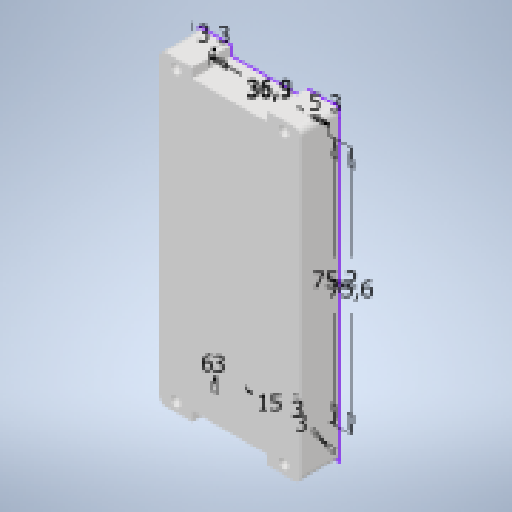
# Autodesk Inventor part: fast_akkum2
Saved by Autodesk Inventor 2023 (Build 270158000, 158)
## iProperties
Created: 2026-02-17
Part Number: fast_akkum2
Material: Типовые
Document SubType Name: Modeling
Designer: garin
Density: 1 g/cm^3
Appearance: По умолчанию
Author: garin
Autodesk Inventor part; units mm, degrees
ref_plane "YZ Plane" through (0, 0, 0) normal (1, 0, 0) x (0, 1, 0)
ref_plane "XZ Plane" through (0, 0, 0) normal (0, 1, 0) x (-1, 0, 0)
ref_plane "XY Plane" through (0, 0, 0) normal (0, 0, 1) x (1, 0, 0)
sketch "Эскиз1" plane through (0, 0, 0) normal (0, 0, 1) x (1, 0, 0)
  line L0 (-18.25, -37.6) -> (18.25, -37.6)
  line L1 (18.25, -37.6) -> (18.25, 37.6)
  line L2 (18.25, 37.6) -> (-18.25, 37.6)
  line L3 (-18.25, 37.6) -> (-18.25, -37.6)
  line L4 (-18.25, 0) -> (18.25, 0) construction
  line L5 (0, 37.6) -> (0, -37.6) construction
  line L6 (-18.45, -37.8) -> (18.45, -37.8)
  line L7 (18.45, -37.8) -> (18.45, 37.8)
  line L8 (18.45, 37.8) -> (-18.45, 37.8)
  line L9 (-18.45, 37.8) -> (-18.45, -37.8)
  line L10 (-7.5, -37.8) -> (7.5, -37.8)
  line L11 (7.5, -37.8) -> (7.5, -40.8)
  line L12 (7.5, -40.8) -> (-7.5, -40.8)
  line L13 (-7.5, -40.8) -> (-7.5, -37.8)
  line L14 (-18.45, -37.8) -> (-18.45, -43.8)
  line L15 (-18.45, -43.8) -> (18.45, -43.8)
  line L16 (18.45, -43.8) -> (18.45, -37.8)
  line L17 (-18.45, 43.8) -> (18.45, 43.8)
  line L18 (-18.45, 37.8) -> (-18.45, 43.8)
  line L19 (18.45, 43.8) -> (18.45, 37.8)
  line L20 (-18.45, -43.8) -> (-21.45, -43.8)
  line L21 (-21.45, -43.8) -> (-21.45, 43.8)
  line L22 (-21.45, 43.8) -> (-18.45, 43.8)
  line L23 (-18.45, 43.8) -> (-18.45, -43.8)
  line L24 (21.45, 43.8) -> (18.45, 43.8)
  line L25 (18.45, 37.8) -> (18.45, 43.8)
  line L26 (18.45, 43.8) -> (18.45, -43.8)
  line L27 (21.45, -43.8) -> (21.45, 43.8)
  line L28 (-7.5, 40.8) -> (-7.5, 37.8)
  line L29 (7.5, 40.8) -> (-7.5, 40.8)
  line L30 (7.5, 37.8) -> (7.5, 40.8)
  line L31 (-21.45, -43.8) -> (-11.45, -43.8)
  line L32 (18.45, -43.8) -> (21.45, -43.8)
  line L33 (21.45, -43.8) -> (11.45, -43.8)
  line L34 (16.45, 46.7) -> (21.45, 46.7)
  line L35 (16.45, 46.7) -> (11.45, 46.7)
  line L36 (11.45, 46.7) -> (11.45, 43.8)
  line L37 (21.45, 46.7) -> (21.45, 43.8)
  line L38 (11.45, 43.8) -> (16.45, 43.8)
  line L39 (-11.45, 46.7) -> (-11.45, 43.8)
  line L40 (-16.45, 46.7) -> (-11.45, 46.7)
  line L41 (-16.45, 46.7) -> (-21.45, 46.7)
  line L42 (-21.45, 46.7) -> (-21.45, 43.8)
  line L43 (-16.45, -46.7) -> (-21.45, -46.7)
  line L44 (-21.45, -46.7) -> (-21.45, -43.8)
  line L45 (-16.45, -46.7) -> (-11.45, -46.7)
  line L46 (-11.45, -46.7) -> (-11.45, -43.8)
  line L47 (11.45, -46.7) -> (11.45, -43.8)
  line L48 (16.45, -46.7) -> (11.45, -46.7)
  line L49 (16.45, -46.7) -> (21.45, -46.7)
  line L50 (21.45, -46.7) -> (21.45, -43.8)
  circle A0 centre (16.45, -43.8) radius 1.5
  circle A1 centre (-16.45, -43.8) radius 1.5
  circle A2 centre (16.45, 43.8) radius 1.5
  circle A3 centre (-16.45, 43.8) radius 1.5
  line L51 (0, 0) -> (-14.3, 0) construction
  line L52 (-14.3, 0) -> (-14.3, 38.8) construction
  line L53 (-14.3, 38.8) -> (0, 38.8) construction
  line L54 (0, 38.8) -> (0, 0) construction
  circle A4 centre (-14.3, 38.8) radius 1.25
  point P0 (-1.9914, -32.8601)
  point P1 (0, -37.8)
  point P2 (-15.05, 37.8)
  point P3 (-13.55, 37.8)
  dimension "d0" = 36.5
  dimension "d1" = 75.2
  dimension "d2" = 36.9
  dimension "d3" = 75.6
  dimension "d4" = 15
  dimension "d5" = 3
  dimension "d6" = 6
  dimension "d7" = 3
  dimension "d8" = 5
  dimension "d10" = 3
  dimension "d11" = 3
  dimension "d12" = 3
  dimension "d13" = 3
  dimension "d19" = 14.3
  dimension "d20" = 38.8
  dimension "d21" = 2.5
  constraints: 110 end point, 20 symmetric about line, 10 parallel, 9 perpendicular, 7 horizontal, 6 midpoint, 6 point on line, 5 centre point, 2 coincident, 2 vertical
  measures "d0" distance of L2.end L1.end
  measures "d1" distance of L1.end L0.end
  measures "d2" distance of L9.start L7.end
  measures "d3" distance of L7.end L7.start
  measures "d4" distance of L11.end L13.start
  measures "d5" distance of L10.end L11.end
  measures "d6" distance of L9.end L23.end
  measures "d7" distance of L21.end L23.start
  measures "d8" distance of L36.end L38.end
  measures "d10" diameter of A0
  measures "d11" diameter of A1
  measures "d12" diameter of A2
  measures "d13" diameter of A3
  measures "d19" distance of L52.end L53.end
  measures "d20" distance of L51.end L52.end
  measures "d21" diameter of A4
extrude "Выдавливание1" add sketch "Эскиз1" along normal blind 12 contours A4 L8 | L8 L18 L17 A3 A2 L19 L30 L29 L28 A4 | L9 L14 L20 L21 L22 L18 | L6 L13 L12 L11 L16 L15 A0 A1 L14 | L22 L42 L41 L40 L39 L17 A3 | L15 A1 L46 L45 L43 L44 L20 | L19 L24 L27 L32 L16 L7 | L17 A2 L36 L35 L34 L37 L24 | L32 L50 L49 L48 L47 L15 A0
fillet "Сопряжение1" radius 2 4 edges at (-21.45, 46.7, 6) (21.45, 46.7, 6) (-21.45, -46.7, 6) (21.45, -46.7, 6)
extrude "Выдавливание3" cut sketch "Эскиз1" against normal blind 10 from surface at 12 contours A4 L8
sketch "Эскиз2" plane through (-11.45, 43.8, 0) normal (0, 1, 0) x (1, 0, 0)
  line L0 (32.9, 0) -> (32.9, -12) construction
  line L1 (32.9, -6) -> (-10, -6) construction
  line L2 (-10, -12) -> (-10, 0) construction
  line L3 (3.95, -12) -> (18.95, -12) construction
  line L4 (11.45, -12) -> (11.45, 0) construction
  line L5 (32.9, -12) -> (30.9, -12) construction
  line L6 (32.9, -12) -> (11.45, -12) construction
  line L7 (11.45, -12) -> (11.45, -9.9) construction
  line L8 (11.45, -9.9) -> (32.9, -9.9) construction
  line L9 (32.9, -9.9) -> (32.9, -12) construction
  circle A0 centre (11.45, -9.9) radius 1.5
  dimension "d24" = 2.1
  dimension "d25" = 3
  constraints: 12 end point, 3 midpoint, 2 parallel, 1 centre point, 1 coincident, 1 horizontal, 1 perpendicular, 1 point on line, 1 vertical
  measures "d24" distance of L6.end L7.end
  measures "d25" diameter of A0
extrude "Выдавливание4" cut sketch "Эскиз2" against normal blind 3
